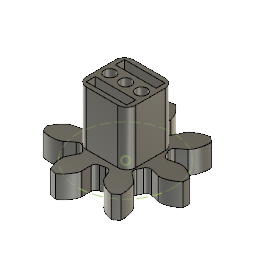
choistepper_gear v2 (Autodesk Fusion 360 design; units mm, degrees)
description: Spur Gear; Module: 3.0; Num Teeth: 7; Pressure Angle: 20.0; Backlash: 0.00 mm
Autodesk Fusion 360 part; units mm, degrees
sketch "Sketch1" plane through (0, 0, 0) normal (0, 0, 1) x (1, 0, 0)
  circle A0 centre (0, 0) radius 11
  line L0 (-4.5, 14) -> (4.5, 14)
  line L1 (4.5, 14) -> (4.5, 12)
  line L2 (4.5, 12) -> (-4.5, 12)
  line L3 (-4.5, 12) -> (-4.5, 14)
  line L4 (0, 0) -> (0, 12)
  line L5 (0, 0) -> (11, 0)
  circle A1 centre (0, 0) radius 15.7054
  line L6 (0, 0) -> (-4.5, 14)
  line L7 (-4.5, 14) -> (-4.806, 14.952)
  line L8 (-8.1423, 9.8971) -> (-12.6423, 2.1029)
  line L9 (-14.3744, 3.1029) -> (-9.8744, 10.8971)
  line L10 (-9.8744, 10.8971) -> (-8.1423, 9.8971)
  line L11 (-12.6423, 2.1029) -> (-14.3744, 3.1029)
  line L12 (-12.6423, -2.1029) -> (-8.1423, -9.8971)
  line L13 (-9.8744, -10.8971) -> (-14.3744, -3.1029)
  line L14 (-14.3744, -3.1029) -> (-12.6423, -2.1029)
  line L15 (-8.1423, -9.8971) -> (-9.8744, -10.8971)
  line L16 (-4.5, -12) -> (4.5, -12)
  line L17 (4.5, -14) -> (-4.5, -14)
  line L18 (-4.5, -14) -> (-4.5, -12)
  line L19 (4.5, -12) -> (4.5, -14)
  line L20 (8.1423, -9.8971) -> (12.6423, -2.1029)
  line L21 (14.3744, -3.1029) -> (9.8744, -10.8971)
  line L22 (9.8744, -10.8971) -> (8.1423, -9.8971)
  line L23 (12.6423, -2.1029) -> (14.3744, -3.1029)
  line L24 (12.6423, 2.1029) -> (8.1423, 9.8971)
  line L25 (9.8744, 10.8971) -> (14.3744, 3.1029)
  line L26 (14.3744, 3.1029) -> (12.6423, 2.1029)
  line L27 (8.1423, 9.8971) -> (9.8744, 10.8971)
  circle A2 centre (0, 0) radius 1.25
  line L28 (-4.5, 4.25) -> (4.5, 4.25)
  line L29 (4.5, 4.25) -> (4.5, 2.25)
  line L30 (4.5, 2.25) -> (-4.5, 2.25)
  line L31 (-4.5, 2.25) -> (-4.5, 4.25)
  line L32 (0, 2.25) -> (0, 4.25)
  line L33 (-3.5, 5.25) -> (3.5, 5.25)
  line L34 (5.5, 3.25) -> (5.5, 0)
  line L35 (5.5, 0) -> (-5.5, 0)
  line L36 (-5.5, 0) -> (-5.5, 3.25)
  arc A3 (-3.5, 5.25) -> (-5.5, 3.25) centre (-3.5, 3.25) ccw
  arc A4 (5.5, 3.25) -> (3.5, 5.25) centre (3.5, 3.25) ccw
  line L37 (-5.5, 0) -> (-5.5, -3.25)
  arc A5 (-5.5, -3.25) -> (-3.5, -5.25) centre (-3.5, -3.25) ccw
  line L38 (-3.5, -5.25) -> (3.5, -5.25)
  arc A6 (3.5, -5.25) -> (5.5, -3.25) centre (3.5, -3.25) ccw
  line L39 (5.5, -3.25) -> (5.5, 0)
  line L40 (4.5, -2.25) -> (-4.5, -2.25)
  line L41 (4.5, -4.25) -> (4.5, -2.25)
  line L42 (-4.5, -4.25) -> (4.5, -4.25)
  line L43 (-4.5, -2.25) -> (-4.5, -4.25)
  circle A7 centre (-3.5, 0) radius 1.25
  circle A8 centre (3.5, 0) radius 1.25
  line L44 (-11, 0) -> (-15.7054, 0)
  circle A9 centre (-13.3527, 0) radius 1.25
  circle A10 centre (6.6764, -11.5638) radius 1.25
  circle A11 centre (6.6764, 11.5638) radius 1.25
  point P0 (0, 11)
  point P1 (0, 12)
  point P2 (0, 1.25)
  point P3 (-2.25, 0)
  point P4 (-1.25, 0)
  dimension "d1" = 9
  dimension "d2" = 2
  dimension "d3" = 90
  dimension "d4" = 1
  dimension "d5" = 1
  dimension "d7" = 360
  dimension "d8" = 11
  dimension "d9" = 2.5
  dimension "d10" = 9
  dimension "d11" = 2
  dimension "d12" = 90
  dimension "d13" = 1
  dimension "d14" = 1
  dimension "d15" = 1
  dimension "d16" = 2
  dimension "d17" = 2
  dimension "d18" = 1
  dimension "d19" = 2.5
  dimension "d20" = 1
  dimension "d34" = 2.5
  dimension "d36" = 360
  constraint coincident A0.centre L4.start
  constraint horizontal L0
  constraint vertical L1
  constraint horizontal L2
  constraint vertical L3
  constraint midpoint L2 P1
  constraint coincident A0 L5.end
  constraint parallel L2 L5
  constraint coincident A0 P0
  constraint coincident L4 P0
  constraint coincident P1 L4.end
  constraint concentric A0 A1
  constraint coincident A1 L7.end
  constraint parallel L6 L7
  constraint concentric A1 A2
  constraint horizontal L28
  constraint vertical L29
  constraint horizontal L30
  constraint vertical L31
  constraint midpoint L30 L32.start
  constraint coincident L4 L32.end
  constraint coincident L28 L32.end
  constraint horizontal L33
  constraint vertical L34
  constraint horizontal L35
  constraint vertical L36
  constraint coincident L5 L34.end
  constraint tangent L33 A3
  constraint tangent L36 A3
  constraint tangent L33 A4
  constraint tangent L34 A4
  constraint symmetric L5 L28.start L42.start
  constraint symmetric L5 L28.end L41.start
  constraint symmetric L5 L29.end L40.start
  constraint symmetric L5 L30.end L40.end
  constraint symmetric L5 L34.end L35.start
  constraint symmetric L5 L35.end L36.start
  constraint symmetric L5 L33.start A5.end
  constraint symmetric L5 L36.end L37.end
  constraint symmetric L5 A3 A5
  constraint symmetric L5 L33.end L38.end
  constraint symmetric L5 L34.start A6.end
  constraint symmetric L5 A4 A6
  constraint coincident A2 P2
  constraint coincident L4 P2
  constraint coincident L35 A7.centre
  constraint coincident A7 P3
  constraint coincident L35 P3
  constraint coincident A2 P4
  constraint coincident L35 P4
  constraint symmetric L4 A7 A8
  constraint coincident A0 L44.start
  constraint coincident A1 L44.end
  constraint horizontal L44
  constraint midpoint L44 A9.centre
  measures "d1" distance of L0.start L0.end
  measures "d2" distance of L0.start L2.end
  measures "d3" angle of L4 L5
  measures "d4" distance of P0 P1
  measures "d5" distance of L0.start L7.end
  measures "d8" distance of A0.centre L5.end
  measures "d9" diameter of A2
  measures "d10" distance of L28.start L28.end
  measures "d11" distance of L28.start L30.end
  measures "d12" angle of L28 L32
  measures "d13" distance of L31 L36
  measures "d14" distance of L28 L33
  measures "d15" distance of L29 L34
  measures "d16" radius of A3
  measures "d17" radius of A4
  measures "d18" distance of L32.start P2
  measures "d19" diameter of A7
  measures "d20" distance of P3 P4
  measures "d34" diameter of A9
extrude "Extrude1" add sketch "Sketch1" along normal blind 9 contours A0 L2 L3 A1 L6 L7 L44 A9 | A0 L0 L1 L2 L4 A1 L7 L44 A9 | A0 L2 L4 L6 | L5 A2 L35 L37 A5 L38 A6 L39 A7 A8 | L4 L5 A2 L28 L29 L30 L33 L34 L35 A4 A8 | L4 L6 L28 L33 | L6 A2 L28 L30 L31 L33 L35 L36 A3 A7 | L4 L6 A2 L30 makes body 1 at (15.6274, -1.5638, 3) makes body 2 at (1.5, -2.25, 3)
sketch "Sketch2" plane through (0, 0, 0) normal (0, 0, -1) x (1, 0, 0)
  line L0 (-12.6423, -2.1029) -> (-8.1423, -9.8971)
  line L1 (-8.1423, -9.8971) -> (-9.8744, -10.8971)
  line L2 (-9.8744, -10.8971) -> (-14.3744, -3.1029)
  line L3 (-14.3744, -3.1029) -> (-12.6423, -2.1029)
  line L4 (8.1423, -9.8971) -> (12.6423, -2.1029)
  line L5 (12.6423, -2.1029) -> (14.3744, -3.1029)
  line L6 (14.3744, -3.1029) -> (9.8744, -10.8971)
  line L7 (9.8744, -10.8971) -> (8.1423, -9.8971)
  line L8 (12.6423, 2.1029) -> (8.1423, 9.8971)
  line L9 (8.1423, 9.8971) -> (9.8744, 10.8971)
  line L10 (9.8744, 10.8971) -> (14.3744, 3.1029)
  line L11 (14.3744, 3.1029) -> (12.6423, 2.1029)
  circle A0 centre (0, 0) radius 11
  line L12 (-8.1423, 9.8971) -> (-12.6423, 2.1029)
  line L13 (-12.6423, 2.1029) -> (-14.3744, 3.1029)
  line L14 (-14.3744, 3.1029) -> (-9.8744, 10.8971)
  line L15 (-9.8744, 10.8971) -> (-8.1423, 9.8971)
  line L16 (4.5, 12) -> (-4.5, 12)
  line L17 (-4.5, 12) -> (-4.5, 14)
  line L18 (-4.5, 14) -> (4.5, 14)
  line L19 (4.5, 14) -> (4.5, 12)
  line L20 (-4.5, -12) -> (4.5, -12)
  line L21 (4.5, -12) -> (4.5, -14)
  line L22 (4.5, -14) -> (-4.5, -14)
  line L23 (-4.5, -14) -> (-4.5, -12)
  circle A1 centre (0, 0) radius 15.7054
  circle A2 centre (0, 0) radius 11
  circle A3 centre (0, 0) radius 15.7054
  circle A4 centre (-13.3527, 0) radius 1.25
  circle A5 centre (6.6764, 11.5638) radius 1.25
  circle A6 centre (6.6764, -11.5638) radius 1.25
  constraint concentric A0 A2
  constraint concentric A0 A3
extrude "Extrude2" add sketch "Sketch2" along normal blind 1 contours L0 L1 L2 L3 | L4 L5 L6 L7 | L8 L9 L10 L11 | L12 L13 L14 L15 | L16 L17 L18 L19 | L20 L21 L22 L23 | A1 A3 | A4 | A5 | A6 bodies 1
sketch "Sketch3" plane through (0, 0, 0) normal (0, 0, -1) x (1, 0, 0)
  line L0 (-4.5, 2.25) -> (-4.5, 4.25)
  line L1 (-4.5, 4.25) -> (4.5, 4.25)
  line L2 (4.5, 4.25) -> (4.5, 2.25)
  line L3 (4.5, 2.25) -> (-4.5, 2.25)
  circle A0 centre (3.5, 0) radius 1.25
  circle A1 centre (-3.5, 0) radius 1.25
  line L4 (-4.5, -2.25) -> (4.5, -2.25)
  line L5 (4.5, -2.25) -> (4.5, -4.25)
  line L6 (4.5, -4.25) -> (-4.5, -4.25)
  line L7 (-4.5, -4.25) -> (-4.5, -2.25)
  circle A2 centre (0, 0) radius 1.25
  line L8 (-5.5, 3.25) -> (-5.5, -3.25)
  arc A3 (-5.5, -3.25) -> (-3.5, -5.25) centre (-4.5, -4.25) ccw
  line L9 (-3.5, -5.25) -> (3.5, -5.25)
  arc A4 (3.5, -5.25) -> (5.5, -3.25) centre (4.5, -4.25) ccw
  line L10 (5.5, -3.25) -> (5.5, 3.25)
  arc A5 (5.5, 3.25) -> (3.5, 5.25) centre (4.5, 4.25) ccw
  line L11 (3.5, 5.25) -> (-3.5, 5.25)
  arc A6 (-3.5, 5.25) -> (-5.5, 3.25) centre (-4.5, 4.25) ccw
  line L12 (-6, 8) -> (6, 8)
  line L13 (6, 8) -> (6, -8)
  line L14 (6, -8) -> (-6, -8)
  line L15 (-6, -8) -> (-6, 8)
  point P0 (-3.5, -3.25)
  point P1 (3.5, -3.25)
  point P2 (3.5, 3.25)
  point P3 (-3.5, 3.25)
  constraint horizontal L12
  constraint vertical L13
  constraint horizontal L14
  constraint vertical L15
extrude "Extrude3" add sketch "Sketch3" along normal blind 1 contours L0 L1 L2 L3 | L4 L5 L6 L7 | L8 A3 L9 A4 L10 A5 L11 A6 bodies 2
sketch "Sketch4" plane through (0, 0, -1) normal (0, 0, -1) x (1, 0, 0)
  circle A0 centre (0, 0) radius 11
  circle A1 centre (0, 0) radius 15.7054
  line L0 (0, 0) -> (12.1661, 12.1661)
  circle A2 centre (12.1661, 12.1661) radius 1.5
  line L1 (0, 0) -> (11, 0)
  circle A3 centre (12.1661, 12.1661) radius 2.5
  line L2 (5.6184, 14.6661) -> (14.047, 14.6661)
  line L3 (14.6661, 5.6184) -> (14.6661, 14.047)
  line L4 (-14.6661, 5.6184) -> (-14.6661, 14.047)
  circle A4 centre (-12.1661, 12.1661) radius 2.5
  line L5 (-5.6184, 14.6661) -> (-14.047, 14.6661)
  circle A5 centre (-12.1661, 12.1661) radius 1.5
  line L6 (-5.6184, -14.6661) -> (-14.047, -14.6661)
  circle A6 centre (-12.1661, -12.1661) radius 2.5
  line L7 (-14.6661, -5.6184) -> (-14.6661, -14.047)
  circle A7 centre (-12.1661, -12.1661) radius 1.5
  line L8 (14.6661, -5.6184) -> (14.6661, -14.047)
  circle A8 centre (12.1661, -12.1661) radius 2.5
  line L9 (5.6184, -14.6661) -> (14.047, -14.6661)
  circle A9 centre (12.1661, -12.1661) radius 1.5
  dimension "d27" = 3
  dimension "d28" = 45
  dimension "d29" = 1
  dimension "d31" = 360
  constraint coincident A0.centre A1.centre
  constraint coincident L0.end A2.centre
  constraint tangent A1 A2
  constraint coincident A0 L1.end
  constraint horizontal L1
  constraint coincident A1 L2.start
  constraint tangent A3 L2
  constraint horizontal L2
  constraint symmetric L0 L2.start L3.start
  constraint symmetric L0 L2.end L3.end
  measures "d27" diameter of A2
  measures "d28" angle of L0 L1
extrude "Extrude4" add sketch "Sketch4" against normal blind 2 contours A1 A3 L3 | A1 L8 A8 | A1 A3 | A1 A8 | A1 A3 L2 | A1 A8 L9 | A1 A4 L5 | A1 L6 A6 | A1 A4 | A1 A6 | A1 L4 A4 | A1 A6 L7 picked at (10.2026, -12.4068) picked at (-10.1946, 12.3655) picked at (-10.1946, -12.3655) bodies 1
extrude "Extrude5" cut 3 faces at (-12.9857, 0.2927, 0) (7.0003, -11.97, 0) (7.0345, 11.8592, 0) along direction (0, 0, -1) blind 3 on bodies 1 bodies 1
extrude "Extrude6" cut 1 faces at (-11.9362, -7.4951, -1) along direction (0, 0, 1) blind 100 on bodies 1 bodies 1
sketch "Sketch1 (2)" plane through (0, 0, 0) normal (0, 0, 1) x (1, 0, 0) in component "Spur Gear (7 teeth)"
  circle A0 centre (0, 0) radius 6.8492
  circle A1 centre (0, 0) radius 0.5
extrude "Extrude1'" add sketch "Sketch1 (2)" along normal blind 3 separate body makes body 3 in component "Spur Gear (7 teeth)"
sketch "Sketch2 (2)" plane through (0, 0, 0) normal (0, 0, 1) x (1, 0, 0) in component "Spur Gear (7 teeth)"
  spline S0 degree 5 poles (9.5856, -2.3387) (9.5963, -2.3413) (9.6179, -2.3461) (9.6504, -2.352) (9.6941, -2.3573) (9.7494, -2.3607) (9.805, -2.3616) (9.8608, -2.3611) (9.9168, -2.3598) (9.9729, -2.3579) (10.0292, -2.3554) (10.0855, -2.352) (10.1419, -2.3475) (10.1985, -2.3418) (10.2552, -2.3349) (10.312, -2.3268) (10.3689, -2.3178) (10.4258, -2.3079) (10.4828, -2.2974) (10.5398, -2.2861) (10.5968, -2.2741) (10.6539, -2.2614) (10.711, -2.2478) (10.7681, -2.2335) (10.8252, -2.2183) (10.8823, -2.2024) (10.9394, -2.1858) (10.9965, -2.1685) (11.0536, -2.1505) (11.1106, -2.1318) (11.1676, -2.1125) (11.2246, -2.0925) (11.2816, -2.0719) (11.3385, -2.0505) (11.3953, -2.0285) (11.4521, -2.0059) (11.5089, -1.9826) (11.5655, -1.9588) (11.6221, -1.9343) (11.6787, -1.9091) (11.7351, -1.8834) (11.7915, -1.8571) (11.8478, -1.8301) (11.904, -1.8026) (11.9601, -1.7745) (12.0162, -1.7458) (12.0721, -1.7165) (12.1279, -1.6867) (12.1836, -1.6562) (12.2392, -1.6252) (12.2947, -1.5937) (12.35, -1.5616) (12.4052, -1.5289) (12.4603, -1.4957) (12.5153, -1.4619) (12.5701, -1.4276) (12.6248, -1.3928) (12.6794, -1.3574) (12.7338, -1.3215) (12.788, -1.285) (12.8422, -1.2481) (12.8961, -1.2106) (12.9499, -1.1726) (13.0035, -1.1341) (13.057, -1.095) (13.1103, -1.0555) (13.1634, -1.0154) (13.2164, -0.9749) (13.2691, -0.9338) (13.3217, -0.8923) (13.3741, -0.8503) (13.4159, -0.8162) (13.4471, -0.7905) (13.4679, -0.7732) (13.4783, -0.7646) knots 0 0 0 0 0 0 0.01428571 0.02857143 0.04285714 0.05714286 0.07142857 0.08571429 0.1 0.11428571 0.12857143 0.14285714 0.15714286 0.17142857 0.18571429 0.2 0.21428571 0.22857143 0.24285714 0.25714286 0.27142857 0.28571429 0.3 0.31428571 0.32857143 0.34285714 0.35714286 0.37142857 0.38571429 0.4 0.41428571 0.42857143 0.44285714 0.45714286 0.47142857 0.48571429 0.5 0.51428571 0.52857143 0.54285714 0.55714286 0.57142857 0.58571429 0.6 0.61428571 0.62857143 0.64285714 0.65714286 0.67142857 0.68571429 0.7 0.71428571 0.72857143 0.74285714 0.75714286 0.77142857 0.78571429 0.8 0.81428571 0.82857143 0.84285714 0.85714286 0.87142857 0.88571429 0.9 0.91428571 0.92857143 0.94285714 0.95714286 0.97142857 0.98571429 1 1 1 1 1 1
  spline S1 degree 5 poles (9.5856, 2.3387) (9.5963, 2.3413) (9.6179, 2.3461) (9.6504, 2.352) (9.6941, 2.3573) (9.7494, 2.3607) (9.805, 2.3616) (9.8608, 2.3611) (9.9168, 2.3598) (9.9729, 2.3579) (10.0292, 2.3554) (10.0855, 2.352) (10.1419, 2.3475) (10.1985, 2.3418) (10.2552, 2.3349) (10.312, 2.3268) (10.3689, 2.3178) (10.4258, 2.3079) (10.4828, 2.2974) (10.5398, 2.2861) (10.5968, 2.2741) (10.6539, 2.2614) (10.711, 2.2478) (10.7681, 2.2335) (10.8252, 2.2183) (10.8823, 2.2024) (10.9394, 2.1858) (10.9965, 2.1685) (11.0536, 2.1505) (11.1106, 2.1318) (11.1676, 2.1125) (11.2246, 2.0925) (11.2816, 2.0719) (11.3385, 2.0505) (11.3953, 2.0285) (11.4521, 2.0059) (11.5089, 1.9826) (11.5655, 1.9588) (11.6221, 1.9343) (11.6787, 1.9091) (11.7351, 1.8834) (11.7915, 1.8571) (11.8478, 1.8301) (11.904, 1.8026) (11.9601, 1.7745) (12.0162, 1.7458) (12.0721, 1.7165) (12.1279, 1.6867) (12.1836, 1.6562) (12.2392, 1.6252) (12.2947, 1.5937) (12.35, 1.5616) (12.4052, 1.5289) (12.4603, 1.4957) (12.5153, 1.4619) (12.5701, 1.4276) (12.6248, 1.3928) (12.6794, 1.3574) (12.7338, 1.3215) (12.788, 1.285) (12.8422, 1.2481) (12.8961, 1.2106) (12.9499, 1.1726) (13.0035, 1.1341) (13.057, 1.095) (13.1103, 1.0555) (13.1634, 1.0154) (13.2164, 0.9749) (13.2691, 0.9338) (13.3217, 0.8923) (13.3741, 0.8503) (13.4159, 0.8162) (13.4471, 0.7905) (13.4679, 0.7732) (13.4783, 0.7646) knots 0 0 0 0 0 0 0.01428571 0.02857143 0.04285714 0.05714286 0.07142857 0.08571429 0.1 0.11428571 0.12857143 0.14285714 0.15714286 0.17142857 0.18571429 0.2 0.21428571 0.22857143 0.24285714 0.25714286 0.27142857 0.28571429 0.3 0.31428571 0.32857143 0.34285714 0.35714286 0.37142857 0.38571429 0.4 0.41428571 0.42857143 0.44285714 0.45714286 0.47142857 0.48571429 0.5 0.51428571 0.52857143 0.54285714 0.55714286 0.57142857 0.58571429 0.6 0.61428571 0.62857143 0.64285714 0.65714286 0.67142857 0.68571429 0.7 0.71428571 0.72857143 0.74285714 0.75714286 0.77142857 0.78571429 0.8 0.81428571 0.82857143 0.84285714 0.85714286 0.87142857 0.88571429 0.9 0.91428571 0.92857143 0.94285714 0.95714286 0.97142857 0.98571429 1 1 1 1 1 1
  arc A0 (13.4783, -0.7646) -> (13.4783, 0.7646) centre (0, 0) ccw
  line L0 (6.6443, -1.6234) -> (9.5856, -2.3387)
  line L1 (6.6443, 1.6234) -> (9.5856, 2.3387)
  line L2 (6.6443, -1.6234) -> (6.6443, 1.6234)
  point P0 (9.8472, -2.3611)
  point P1 (10.1166, -2.3494)
  point P2 (10.3908, -2.3139)
  point P3 (10.6685, -2.2578)
  point P4 (10.9489, -2.1828)
  point P5 (11.2311, -2.09)
  point P6 (11.5144, -1.9802)
  point P7 (11.7982, -1.8538)
  point P8 (12.0818, -1.7112)
  point P9 (12.3648, -1.5527)
  point P10 (12.6465, -1.3786)
  point P11 (12.9264, -1.1891)
  point P12 (13.2038, -0.9844)
  point P13 (9.8472, 2.3611)
  point P14 (10.1166, 2.3494)
  point P15 (10.3908, 2.3139)
  point P16 (10.6685, 2.2578)
  point P17 (10.9489, 2.1828)
  point P18 (11.2311, 2.09)
  point P19 (11.5144, 1.9802)
  point P20 (11.7982, 1.8538)
  point P21 (12.0818, 1.7112)
  point P22 (12.3648, 1.5527)
  point P23 (12.6465, 1.3786)
  point P24 (12.9264, 1.1891)
  point P25 (13.2038, 0.9844)
extrude "Extrude2'" add sketch "Sketch2 (2)" along normal blind 3 bodies 3 in component "Spur Gear (7 teeth)"
fillet "Fillet1" radius 1 2 edges at (6.6535, -1.6257, 1.5) (6.6535, 1.6257, 1.5) on bodies 3 in component "Spur Gear (7 teeth)"
pattern_circular "C-Pattern1" count 7 over 360 about axis through (0, 0, 0) along (0, 0, 1) of "Extrude2'", "Fillet1" in component "Spur Gear (7 teeth)"
sketch "Sketch3 (2)" plane through (0, 0, 0) normal (0, 0, 1) x (1, 0, 0) in component "Spur Gear (7 teeth)"
  circle A0 centre (0, 0) radius 10.5 construction
extrude "Extrude3'" add 1 faces at (2.8195, -3.5355, 0) along direction (0, 0, -1) blind 2 on bodies 3 bodies 3 in component "Spur Gear (7 teeth)"
extrude "Extrude7" add 1 faces at (0.0311, -1.9155, 9) along direction (0, 0, 1) blind 2 on bodies 2 bodies 2 1
extrude "Extrude8" cut 4 faces at (-5.0812, 4.8811, 0) (5.0812, 4.8811, 0) (-5.1311, -4.8312, 0) (5.1311, -4.8312, 0) along direction (0, 0, 1) up to surface end surface through (0, 0, -1) normal (0, 0, 1) offset 0 on bodies 2 bodies 2
component "Spur Gear (7 teeth)" placed x (1, 0, 0) y (0, 1, 0) z (0, 0, 1) at (0, 0, -4)
